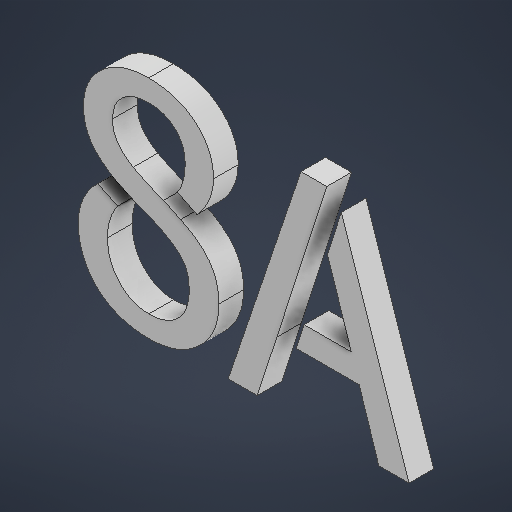
# Autodesk Inventor part: 8А встав
Saved by Autodesk Inventor 2025 (Build 290162000, 162)
## iProperties
Created: 2025-01-14
Part Number: 8А встав
Material: Типовые
Document SubType Name: Modeling
Designer: Phantom
Density: 1 g/cm^3
Appearance: По умолчанию
Author: Phantom
Autodesk Inventor part; units mm, degrees
ref_plane "YZ Plane" through (0, 0, 0) normal (1, 0, 0) x (0, 1, 0)
ref_plane "XZ Plane" through (0, 0, 0) normal (0, 1, 0) x (-1, 0, 0)
ref_plane "XY Plane" through (0, 0, 0) normal (0, 0, 1) x (1, 0, 0)
sketch "Эскиз1" plane through (0, 0, 0) normal (0, 0, 1) x (1, 0, 0)
  line L0 (12.5971, -3.2747) -> (20.2523, -3.2747)
  line L1 (20.2523, -3.2747) -> (16.3816, 8.4993)
  line L2 (16.3816, 8.4993) -> (18.6385, 15.5206)
  line L3 (18.6385, 15.5206) -> (29.6121, -17.0308)
  line L4 (29.6121, -17.0308) -> (24.7053, -17.0308)
  line L5 (24.7053, -17.0308) -> (21.5286, -7.2456)
  line L6 (21.5286, -7.2456) -> (11.3208, -7.2456)
  line L7 (11.3208, -7.2456) -> (12.5971, -3.2747)
  line L8 (16.2744, 17.9692) -> (8.1696, -7.2456)
  line L9 (8.1696, -7.2456) -> (4.993, -17.0308)
  line L10 (4.993, -17.0308) -> (0.2847, -17.0308)
  line L11 (0.2847, -17.0308) -> (12.0837, 17.9692)
  line L12 (12.0837, 17.9692) -> (16.2744, 17.9692)
  spline S0 degree 2 poles (-6.6926, 9.8006) (-6.6926, 12.1548) (-9.8409, 15.3031) (-12.6488, 15.3031) knots 0 0 0 1 2 2 2
  spline S1 degree 2 poles (-12.6488, 15.3031) (-15.2015, 15.3031) (-18.4633, 12.4951) (-18.4633, 10.0843) knots 0 0 0 1 2 2 2
  spline S2 degree 2 poles (-18.4633, 10.0843) (-18.4633, 8.3541) (-16.7898, 5.9432) (-15.1164, 4.9789) knots 0 0 0 1 2 2 2
  spline S3 degree 2 poles (-15.1164, 4.9789) (-14.4074, 4.5818) (-11.4009, 3.192) (-10.1813, 2.7949) knots 0 0 0 1 2 2 2
  line L13 (-10.1813, 2.7949) -> (-7.43, 1.4619)
  spline S4 degree 2 poles (-7.43, 1.4619) (-4.3668, 0.0437) (-1.2185, -4.0405) (-1.2185, -7.2739) knots 0 0 0 1 2 2 2
  spline S5 degree 2 poles (-1.2185, -7.2739) (-1.2185, -11.7553) (-7.742, -17.825) (-12.6205, -17.825) knots 0 0 0 1 2 2 2
  spline S6 degree 2 poles (-12.6205, -17.825) (-15.2299, -17.825) (-19.5127, -16.265) (-21.0159, -14.8185) knots 0 0 0 1 2 2 2
  spline S7 degree 2 poles (-21.0159, -14.8185) (-22.4908, -13.4004) (-24.0224, -9.543) (-24.0224, -7.359) knots 0 0 0 1 2 2 2
  spline S8 degree 2 poles (-24.0224, -7.359) (-24.0224, -4.5227) (-21.8258, -1.0738) (-20.871, -0.2006) knots 0 0 0 1 1.44761 1.44761 1.44761
  line L14 (-20.871, -0.2006) -> (-17.6341, -1.7373)
  spline S9 degree 2 poles (-17.6341, -1.7373) (-17.9742, -2.2001) (-19.2858, -4.6078) (-19.2858, -7.0187) knots 0.733023 0.733023 0.733023 1 2 2 2
  spline S10 degree 2 poles (-19.2858, -7.0187) (-19.2858, -10.1953) (-15.4568, -14.3363) (-12.5638, -14.3363) knots 0 0 0 1 2 2 2
  spline S11 degree 2 poles (-12.5638, -14.3363) (-9.614, -14.3363) (-6.0403, -10.791) (-6.0403, -7.7277) knots 0 0 0 1 2 2 2
  spline S12 degree 2 poles (-6.0403, -7.7277) (-6.0403, -5.5722) (-7.742, -3.0195) (-10.1529, -1.7148) knots 0 0 0 1 2 2 2
  spline S13 degree 2 poles (-10.1529, -1.7148) (-10.9471, -1.261) (-13.6132, -0.2115) (-15.2866, 0.4692) knots 0 0 0 1 2 2 2
  line L15 (-15.2866, 0.4692) -> (-18.0945, 1.8022)
  spline S14 degree 2 poles (-18.0945, 1.8022) (-20.6756, 3.3055) (-23.1715, 6.8792) (-23.1715, 9.5454) knots 0 0 0 1 2 2 2
  spline S15 degree 2 poles (-23.1715, 9.5454) (-23.1715, 13.4878) (-17.2153, 18.7633) (-12.6205, 18.7633) knots 0 0 0 1 2 2 2
  spline S16 degree 2 poles (-12.6205, 18.7633) (-7.8555, 18.7633) (-2.0978, 13.7714) (-2.0978, 9.8573) knots 0 0 0 1 2 2 2
  spline S17 degree 2 poles (-2.0978, 9.8573) (-2.0978, 7.5032) (-4.029, 4.278) (-4.7812, 3.512) knots 0 0 0 1 1.403871 1.403871 1.403871
  line L16 (-4.7812, 3.512) -> (-7.9537, 5.0492)
  spline S18 degree 2 poles (-7.9537, 5.0492) (-7.628, 5.5274) (-6.6926, 7.6734) (-6.6926, 9.8006) knots 0.706651 0.706651 0.706651 1 2 2 2
  point P0 (0, 0)
  point P1 (1.7035, -0.9566)
  point P2 (1.7035, -0.9566)
  constraints: 34 end point, 57 other
extrude "Выдавливание1" add sketch "Эскиз1" along normal blind 4
